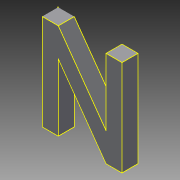
# Autodesk Inventor part: inventor N
Saved by Autodesk Inventor 2013 (Build 170138000, 138)
## iProperties
Created: 2014-03-22
Part Number: inventor N
Material: Generic
Document SubType Name: Modeling
Designer: kahohbein
Density: 1 g/cm^3
Author: kahohbein
Autodesk Inventor part; units mm, degrees
ref_plane "YZ Plane" through (0, 0, 0) normal (1, 0, 0) x (0, 1, 0)
ref_plane "XZ Plane" through (0, 0, 0) normal (0, 1, 0) x (-1, 0, 0)
ref_plane "XY Plane" through (0, 0, 0) normal (0, 0, 1) x (1, 0, 0)
sketch "Sketch1" plane through (0, 0, 0) normal (0, 0, 1) x (1, 0, 0)
  line L0 (508, 0) -> (508, 609.6)
  line L1 (0, 609.6) -> (0, 0)
  line L2 (0, 609.6) -> (101.6, 609.6)
  line L3 (508, 609.6) -> (406.4, 609.6)
  line L4 (406.4, 609.6) -> (406.4, 244.5435)
  line L5 (508, 0) -> (406.4, 0)
  line L6 (0, 0) -> (101.6, 0)
  line L7 (101.6, 0) -> (101.6, 365.0565)
  line L8 (0, 0) -> (101.6, 0)
  line L9 (406.4, 0) -> (508, 0)
  line L10 (508, 609.6) -> (406.4, 609.6)
  line L11 (101.6, 609.6) -> (0, 609.6)
  line L12 (406.4, 244.5435) -> (406.4, 182.5282)
  line L13 (406.4, 182.5282) -> (101.6, 609.6)
  line L14 (406.4, 0) -> (101.6, 427.0718)
  line L15 (101.6, 427.0718) -> (101.6, 345.8678)
  dimension "d0" = 508
  dimension "d1" = 609.6
  dimension "d2" = 101.6
  dimension "d3" = 101.6
  dimension "d4" = 101.6
  dimension "d5" = 101.6
  constraints: 32 end point, 7 parallel, 5 perpendicular, 2 horizontal, 1 point on line
  measures "d0" distance of L1.start L0.end
  measures "d1" distance of L0.end L0.start
  measures "d2" distance of L1.start L2.end
  measures "d3" distance of L0.end L3.end
  measures "d4" distance of L0.start L5.end
  measures "d5" distance of L1.end L6.end
extrude "Extrusion1" add sketch "Sketch1" along normal blind 101.6
sketch "Sketch2" plane through (0, 0, 101.6) normal (0, 0, 1) x (1, 0, 0)
  line L0 (0, 0) -> (101.6, 0) projected
  line L1 (101.6, 0) -> (101.6, 427.0718) projected
  line L2 (101.6, 427.0718) -> (406.4, 0) projected
  line L3 (406.4, 0) -> (508, 0) projected
  line L4 (508, 0) -> (508, 609.6) projected
  line L5 (508, 609.6) -> (406.4, 609.6) projected
  line L6 (406.4, 609.6) -> (406.4, 182.5282) projected
  line L7 (406.4, 182.5282) -> (101.6, 609.6) projected
  line L8 (101.6, 609.6) -> (0, 609.6) projected
  line L9 (0, 609.6) -> (0, 0) projected
sketch "Sketch3" plane through (508, 0, 0) normal (1, 0, 0) x (0, 0, -1)
  line L0 (0, 0) -> (0, 609.6) projected
  line L1 (0, 609.6) -> (-101.6, 609.6) projected
  line L2 (-101.6, 0) -> (-101.6, 609.6) projected
  line L3 (0, 0) -> (-101.6, 0) projected
sketch "Sketch4" plane through (406.4, 609.6, 0) normal (0, 1, 0) x (1, 0, 0)
  line L0 (101.6, 0) -> (0, 0) projected
  line L1 (0, 0) -> (0, -101.6) projected
  line L2 (101.6, -101.6) -> (0, -101.6) projected
  line L3 (101.6, 0) -> (101.6, -101.6) projected
  point P0 (-406.4, 0)
sketch "Sketch5" plane through (101.6, 609.6, 101.6) normal (0.8139599, 0.5809211, 0) x (0, 0, -1)
  line L0 (101.6, -524.684) -> (101.6, 0) projected
  line L1 (101.6, 0) -> (0, 0) projected
  line L2 (0, -524.684) -> (0, 0) projected
  line L3 (101.6, -524.684) -> (0, -524.684) projected
  point P0 (101.6, -437.1684)
sketch "Sketch6" plane through (101.6, 0, 0) normal (1, 0, 0) x (0, 0, -1)
  line L0 (0, 0) -> (0, 427.0718) projected
  line L1 (0, 427.0718) -> (-101.6, 427.0718) projected
  line L2 (-101.6, 0) -> (-101.6, 427.0718) projected
  line L3 (0, 0) -> (-101.6, 0) projected
body "Solid1"
